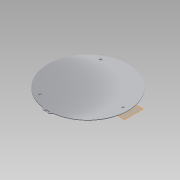
# Autodesk Inventor part: Part21
Saved by Autodesk Inventor 2014 (Build 180170000, 170)
## iProperties
Created: 2016-03-29
Part Number: Part21
Material: Aluminum 6061
Document SubType Name: Modeling
Designer: admin
Density: 2.71 g/cm^3
Appearance: Aluminum - Flat
Mass: 243.544 g
Surface Area: 1014.44 cm^2
Volume: 89.8686 cm^3
Author: admin
Autodesk Inventor part; units mm, degrees
ref_plane "YZ Plane" through (0, 0, 0) normal (1, 0, 0) x (0, 1, 0)
ref_plane "XZ Plane" through (0, 0, 0) normal (0, 1, 0) x (-1, 0, 0)
ref_plane "XY Plane" through (0, 0, 0) normal (0, 0, 1) x (1, 0, 0)
ref_plane "Work Plane1" through (0, 0, 0) normal (0, 0, 1) x (1, 0, 0)
sketch "Sketch1" plane through (0, 0, 0) normal (0, 0, 1) x (1, 0, 0)
  circle A0 centre (-115, 0) radius 5 projected
  circle A1 centre (-115, 0) radius 126
  point P0 (0, 0)
  dimension "d0" = 252
  constraints: 1 centre point, 1 coincident
  measures "d0" diameter of A1
extrude "Extrusion1" add sketch "Sketch1" along normal blind 1.8 contours A0 | A1
sketch "Sketch2" plane through (-115, 0, 1.8) normal (0, 0, 1) x (1, 0, 0)
  circle A0 centre (-55, 95.2628) radius 1.6
  circle A1 centre (-55, -95.2628) radius 1.75
  circle A2 centre (110, 0) radius 1.6
  circle A3 centre (0, 0) radius 126 projected
  line L0 (-55, 95.2628) -> (110, 0)
  line L1 (110, 0) -> (-55, -95.2628)
  line L2 (-55, -95.2628) -> (-55, 95.2628)
  point P0 (115, 0)
  dimension "d3" = 3.2
  dimension "d4" = 3.5
  dimension "d5" = 3.2
  dimension "d11" = 110
  constraints: 6 end point, 3 centre point, 3 coincident, 7 other
  measures "d3" diameter of A0
  measures "d4" diameter of A1
  measures "d5" diameter of A2
  measures "d11" distance of A2.centre A3.centre
extrude "Extrusion2" cut sketch "Sketch2" against normal blind 10 contours A0 L0 L2 | L2 L0 A0 | L2 L1 A1 | A1 L1 L2 | L0 L1 A2 | A2 L1 L0
chamfer "Chamfer1" distance 1.7 angle 45 3 edges at (-6.6, 0, 1.8) (-171.6, 95.2628, 1.8) (-171.75, -95.2628, 1.8)
sketch "Sketch3" plane through (-115, 0, 1.8) normal (0, 0, 1) x (1, 0, 0)
  circle A0 centre (0, 0) radius 126 projected
  line L0 (-1, -129) -> (-5.9628, -131.8653)
  line L1 (1, -129) -> (5.9628, -131.8653)
  arc A1 (6.0472, -127.8571) -> (5.9528, -125.8593) centre (6, -126.8582) ccw
  arc A2 (-5.9528, -125.8593) -> (-6.0472, -127.8571) centre (-6, -126.8582) ccw
  line L2 (13.7031, -128.2781) -> (16.5283, -124.9112)
  line L3 (-13.7031, -128.2781) -> (-16.5283, -124.9112)
  arc A3 (-6.538, -131.838) -> (-5.9628, -131.8653) centre (0, 0) ccw
  arc A4 (5.9628, -131.8653) -> (6.538, -131.838) centre (0, 0) ccw
  line L4 (1, -127.9961) -> (1, -129)
  line L5 (-1, -127.9961) -> (-1, -129)
  arc A5 (-6.0472, -127.8571) -> (-1, -127.9961) centre (0, 0) ccw
  arc A6 (1, -127.9961) -> (6.0472, -127.8571) centre (0, 0) ccw
  arc A7 (-13.7031, -128.2781) -> (-6.538, -131.838) centre (-6.0427, -121.8503) ccw
  arc A8 (6.538, -131.838) -> (13.7031, -128.2781) centre (6.0427, -121.8503) ccw
  point P0 (115, 0)
  point P1 (10.9628, -131.544)
  point P2 (-10.9628, -131.544)
  dimension "d17" = 129
  dimension "d18" = 129
  dimension "d23" = 5
  dimension "d25" = 5
  dimension "d28" = 10
  constraints: 22 point on circle, 12 end point, 8 centre point, 6 tangent, 2 point on line, 1 coincident, 1 equal radius
  measures "d17" vertical distance of A3.centre L1.start
  measures "d18" vertical distance of A3.centre L0.start
  measures "d23" horizontal distance of L1.end point (10.963, -131.544)
  measures "d25" horizontal distance of L0.end point (-10.963, -131.544)
  measures "d28" radius of A7
extrude "Extrusion3" add sketch "Sketch3" against normal up to surface (1.8 mm away) contours A0 A2 A5 L5 L0 A3 A7 L3 | L2 A8 A4 L1 L4 A6 A1 A0
fillet "Fillet1" radius 5 4 edges at (-109.0372, -131.8653, 0.9) (-120.9628, -131.8653, 0.9) (-131.5283, -124.9112, 0.9) (-98.4717, -124.9112, 0.9)
sketch "Sketch4" plane through (0, 0, 0) normal (0, 0, -1) x (-1, 0, 0)
  arc A0 (133.3939, -124.6502) -> (96.6061, -124.6502) centre (115, 0) ccw projected
  arc A1 (116, -127.9961) -> (121.0472, -127.8571) centre (115, 0) ccw projected
  line L0 (115, 0) -> (252.9222, 0) construction
  line L1 (209.3241, 52.4043) -> (223.0286, 58.5024)
  line L2 (229.1267, 44.7979) -> (215.4222, 38.6998)
  line L3 (209.3241, 52.4043) -> (229.1267, 44.7979) construction
  line L4 (223.0286, 58.5024) -> (215.4222, 38.6998) construction
  line L5 (211.6138, 47.2585) -> (225.2106, 53.5988)
  line L6 (223.0286, 58.5024) -> (225.2106, 53.5988)
  line L7 (226.0238, 51.7712) -> (229.1267, 44.7979)
  line L8 (215.4222, 38.6998) -> (212.427, 45.431)
  line L9 (211.6138, 47.2585) -> (209.3241, 52.4043)
  line L10 (115, 0) -> (226.0238, 51.7712)
  point P0 (0, 0)
  point P1 (219.2254, 48.6011)
  dimension "d34" = 15
  dimension "d36" = 115
  constraints: 22 end point, 6 parallel, 2 midpoint, 2 perpendicular, 2 point on line, 1 horizontal
  measures "d34" distance between parallel lines of L2 L1
  measures "d36" distance of A0.centre point (219.225, 48.601)
extrude "Extrusion4" add sketch "Sketch4" along normal blind 1
body "Solid1"
